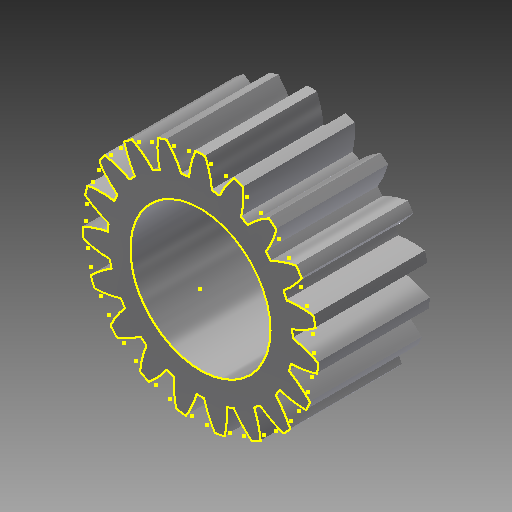
# Autodesk Inventor part: Spur Gear1
Saved by Autodesk Inventor 2017 (Build 210142000, 142)
## iProperties
Created: 2019-09-07
Part Number: Spur Gear1
Material: Steel
Document SubType Name: Modeling
Designer: Dell
Categories: <?xml version="1.0" encoding="UTF-16"?> <MemberInstance><Categories><FamilyTemplate><FamilyTemplateParameter ValueType="xs:double" Id="1" ObjectReferenceKey="da_z" ObjectType="kUserParameterObject"/><FamilyTemplateParameter ValueType="xs:double" Id="2" ObjectReferenceKey="da_b" ObjectType="kUserParameterObject"/><FamilyTemplateParameter ValueType="xs:double" Id="3" ObjectReferenceKey="da_beta" ObjectType="kUserParameterObject"/><FamilyTemplateParameter ValueType="xs:double" Id="4" ObjectReferenceKey="da_da" ObjectType="kUserParameterObject"/><FamilyTemplateParameter ValueType="xs:double" Id="5" ObjectReferenceKey="da_aw" ObjectType="kUserParameterObject"/><FamilyTemplateParameter ValueType="xs:string" Id="6" ObjectReferenceKey="EAIAABAAAACIAQAAAAAAAIAAAAAAAAAA" ObjectType="83910656" SubObjectId="SurfaceGeometry"/></FamilyTemplate><ParamToTemplateMap><ParamToTemplate CategoryParameter="//CategoryParameter[@InternalName='046C89C9-8512-4d59-83FE-43B91F4F132A']" TemplateParameter="1"/><ParamToTemplate CategoryParameter="//CategoryParameter[@InternalName='2552DF32-E462-4b46-AEBF-C6C7768E72AC']" TemplateParameter="2"/><ParamToTemplate CategoryParameter="//CategoryParameter[@InternalName='C9EE641D-15FC-4fae-A226-E94C4372FDD7']" TemplateParameter="3"/><ParamToTemplate><ParamToTemplate CategoryParameter="//CategoryParameter[@InternalName='00B6519A-459B-49c7-AD84-2E56D39A5744']" ConstantValue="0.000000"/></ParamToTemplate><ParamToTemplate><ParamToTemplate CategoryParameter="//CategoryParameter[@InternalName='04B31F0E-C7A6-4894-AA32-9629BEFACF47']" ConstantValue="1.000000"/></ParamToTemplate><ParamToTemplate><ParamToTemplate CategoryParameter="//CategoryParameter[@InternalName='43CBEC2E-7847-49e7-A936-2F7889FCB2D9']" ConstantValue="0.250000"/></ParamToTemplate><ParamToTemplate><ParamToTemplate CategoryParameter="//CategoryParameter[@InternalName='B1EFC894-105D-4ebd-86BF-FA20ED196853']" ConstantValue="0.350000"/></ParamToTemplate><ParamToTemplate><ParamToTemplate CategoryParameter="//CategoryParameter[@InternalName='51175063-3D10-4879-93E8-6246FE8B403D']" ConstantValue="2060000000.000000"/></ParamToTemplate><ParamToTemplate><ParamToTemplate CategoryParameter="//CategoryParameter[@InternalName='A3A52E27-4454-46a9-B0BD-C932399B70AF']" ConstantValue="0.300000"/></ParamToTemplate><ParamToTemplate><ParamToTemplate CategoryParameter="//CategoryParameter[@InternalName='91B76062-C214-41d9-B1B9-14D2AB99603D']" ConstantValue="0.200000"/></ParamToTemplate><ParamToTemplate><ParamToTemplate CategoryParameter="//CategoryParameter[@InternalName='374E806E-8B8A-4dda-A9AA-1039D6500AD2']" ConstantValue="5.000000"/></ParamToTemplate><ParamToTemplate><ParamToTemplate CategoryParameter="//CategoryParameter[@InternalName='2D373A89-B862-43d6-8D0B-0CBF12AB9F6C']" ConstantValue="0.392699"/></ParamToTemplate><ParamToTemplate CategoryParameter="//CategoryParameter[@InternalName='37777632-D6A2-4fac-9D53-DB8ACD95C989']" TemplateParameter="4"/><ParamToTemplate CategoryParameter="//CategoryParameter[@InternalName='FD1017F1-B727-4f7e-9707-0F86F1FF9423']" TemplateParameter="5"/><ParamToTemplate><ParamToTemplate CategoryParameter="//CategoryParameter[@InternalName='9E1B4470-B2D3-4ff1-B813-535BB4CDF51A']" ConstantValue="3520000.000000"/></ParamToTemplate><ParamToTemplate><ParamToTemplate CategoryParameter="//CategoryParameter[@InternalName='F8452263-BFF6-458c-9FB1-07C4B99E95CD']" ConstantValue="11400000.000000"/></ParamToTemplate><ParamToTemplate><ParamToTemplate CategoryParameter="//CategoryParameter[@InternalName='3E3BB259-FD49-497f-8171-6EBC954A3479']" ConstantValue="2.000000"/></ParamToTemplate><ParamToTemplate CategoryParameter="//CategoryParameter[@InternalName='27C3BAF2-7550-4e4b-AE2C-0DB134B7D9B7']" TemplateParameter="6"/></ParamToTemplateMap><Category DisplayName="Gear" InternalName="DC85795E-93AB-48d5-8EEE-5A27447B64BD" Mnemonic="Gear"><CategoryParameter DisplayName="z" InternalName="046C89C9-8512-4d59-83FE-43B91F4F132A" Mnemonic="z"/><CategoryParameter DisplayName="b" InternalName="2552DF32-E462-4b46-AEBF-C6C7768E72AC" Mnemonic="b"/><CategoryParameter DisplayName="||b|" InternalName="C9EE641D-15FC-4fae-A226-E94C4372FDD7" Mnemonic="beta"/><CategoryParameter DisplayName="x" InternalName="00B6519A-459B-49c7-AD84-2E56D39A5744" Mnemonic="x"/><CategoryParameter DisplayName="a*" InternalName="04B31F0E-C7A6-4894-AA32-9629BEFACF47" Mnemonic="a"/><CategoryParameter DisplayName="c*" InternalName="43CBEC2E-7847-49e7-A936-2F7889FCB2D9" Mnemonic="c"/><CategoryParameter DisplayName="r|.f|*" InternalName="B1EFC894-105D-4ebd-86BF-FA20ED196853" Mnemonic="rf"/><CategoryParameter DisplayName="E" InternalName="51175063-3D10-4879-93E8-6246FE8B403D" Mnemonic="E"/><CategoryParameter DisplayName="||m|" InternalName="A3A52E27-4454-46a9-B0BD-C932399B70AF" Mnemonic="mi"/><Category DisplayName="SpurGear" InternalName="26C5A22E-A91E-4dfd-A3B3-23CCAFAE1764" Mnemonic="SpurGear"><CategoryParameter DisplayName="m" InternalName="91B76062-C214-41d9-B1B9-14D2AB99603D" Mnemonic="m"/><CategoryParameter DisplayName="P" InternalName="374E806E-8B8A-4dda-A9AA-1039D6500AD2" Mnemonic="PP"/><CategoryParameter DisplayName="||a|" InternalName="2D373A89-B862-43d6-8D0B-0CBF12AB9F6C" Mnemonic="alpha"/><CategoryParameter DisplayName="d|.a|" InternalName="37777632-D6A2-4fac-9D53-DB8ACD95C989" Mnemonic="da"/><CategoryParameter DisplayName="a|.w|" InternalName="FD1017F1-B727-4f7e-9707-0F86F1FF9423" Mnemonic="aw"/><CategoryParameter DisplayName="||s||.Flim|" InternalName="9E1B4470-B2D3-4ff1-B813-535BB4CDF51A" Mnemonic="sFlim"/><CategoryParameter DisplayName="||s||.Hlim|" InternalName="F8452263-BFF6-458c-9FB1-07C4B99E95CD" Mnemonic="sHlim"/><CategoryParameter DisplayName="type" InternalName="3E3BB259-FD49-497f-8171-6EBC954A3479" Mnemonic="type"/><CategoryParameter DisplayName="PitchDiameter" InternalName="27C3BAF2-7550-4e4b-AE2C-0DB134B7D9B7" Mnemonic="IDS_PITCHDIAM"/></Category></Category></Categories></MemberInstance>
Density: 1 g/cm^3
Appearance: Steel
CustomPartVersion: 1
Author: Dell
Autodesk Inventor part; units mm, degrees
ref_plane "YZ Plane" through (0, 0, 0) normal (1, 0, 0) x (0, 1, 0)
ref_plane "XZ Plane" through (0, 0, 0) normal (0, 1, 0) x (-1, 0, 0)
ref_plane "XY Plane" through (0, 0, 0) normal (0, 0, 1) x (1, 0, 0)
sketch "Sketch1" plane through (0, 0, 0) normal (0, 0, 1) x (1, 0, 0)
  circle A0 centre (0, 0) radius 21
  dimension "d0" = 42
  constraints: 1 centre point
  measures "d0" diameter of A0
extrude "Extrusion1" add sketch "Sketch1" along normal blind 20
ref_plane "Work Plane2" through (0, 0, 10) normal (0, 0, 1) x (1, 0, 0)
sketch "Sketch2" plane through (0, 0, 0) normal (0, 0, -1) x (-1, 0, 0)
  circle A0 centre (0, 0) radius 21 projected
  circle A1 centre (0, 0) radius 19
  dimension "d3" = 38
  constraints: 1 centre point, 1 coincident
  measures "d3" diameter of A1
surface extrude "Pitch Diameter" sketch "Sketch2" against normal through all shown no curves A1
ref_plane "Work Plane8" through (0, 0, 0) normal (0.9863613, 0.1645946, 0) x (0, 0, 1)
ref_plane "Work Plane9" through (0, 0, 0) normal (1, 0, 0) x (0, 1, 0)
spur gear teeth "Spur Gear" teeth 19 pitch diameter 38 tip diameter 42 root diameter 33 face width 20 start plane through (0, 0, 0) normal (0, 0, -1) x (-1, 0, 0)
sketch "Sketch3" plane through (0, 0, 20) normal (0, 0, 1) x (1, 0, 0)
  circle A0 centre (0, 0) radius 12.5
  dimension "d49" = 25
  constraints: 1 centre point, 1 coincident
  measures "d49" diameter of A0
extrude "Extrusion2" cut sketch "Sketch3" against normal through all
sketch "Sketch4" plane through (0, 0, 20) normal (0, 0, 1) x (1, 0, 0)
  circle A0 centre (0, 0) radius 12.5 projected
  arc A1 (-7.6337, 19.5634) -> (-7.2467, 14.8235) centre (8.4724, 18.4924) ccw projected
  arc A2 (-7.2467, 14.8235) -> (-8.4461, 14.1744) centre (0, 0) ccw projected
  arc A3 (-8.4461, 14.1744) -> (-12.2026, 17.0908) centre (-20.1151, 3.0216) ccw projected
  arc A4 (-12.2026, 17.0908) -> (-13.5723, 16.0248) centre (0, 0) ccw projected
  arc A5 (-13.5723, 16.0248) -> (-11.6673, 11.6673) centre (2.0089, 20.2414) ccw projected
  arc A6 (-11.6673, 11.6673) -> (-12.5909, 10.6639) centre (0, 0) ccw projected
  arc A7 (-12.5909, 10.6639) -> (-17.0908, 12.2026) centre (-20.0064, -3.6735) ccw projected
  arc A8 (-17.0908, 12.2026) -> (-18.0401, 10.7496) centre (0, 0) ccw projected
  arc A9 (-18.0401, 10.7496) -> (-14.8235, 7.2467) centre (-4.6724, 19.7969) ccw projected
  arc A10 (-14.8235, 7.2467) -> (-15.3713, 5.9979) centre (0, 0) ccw projected
  arc A11 (-15.3713, 5.9979) -> (-20.127, 5.9921) centre (-17.7296, -9.9705) ccw projected
  arc A12 (-20.127, 5.9921) -> (-20.5531, 4.3095) centre (0, 0) ccw projected
  arc A13 (-20.5531, 4.3095) -> (-16.3733, 2.0409) centre (-10.8472, 17.2072) ccw projected
  arc A14 (-16.3733, 2.0409) -> (-16.4859, 0.6819) centre (0, 0) ccw projected
  arc A15 (-16.4859, 0.6819) -> (-20.9821, -0.8678) centre (-13.5315, -15.1871) ccw projected
  arc A16 (-20.9821, -0.8678) -> (-20.8387, -2.5975) centre (0, 0) ccw projected
  arc A17 (-20.8387, -2.5975) -> (-16.1488, -3.3861) centre (-15.8467, 12.7527) ccw projected
  arc A18 (-16.1488, -3.3861) -> (-15.8141, -4.708) centre (0, 0) ccw projected
  arc A19 (-15.8141, -4.708) -> (-19.5634, -7.6337) centre (-7.8671, -18.7579) ccw projected
  arc A20 (-19.5634, -7.6337) -> (-18.8662, -9.2231) centre (0, 0) ccw projected
  arc A21 (-18.8662, -9.2231) -> (-14.1744, -8.4461) centre (-19.1289, 6.9163) ccw projected
  arc A22 (-14.1744, -8.4461) -> (-13.4285, -9.5878) centre (0, 0) ccw projected
  arc A23 (-13.4285, -9.5878) -> (-16.0248, -13.5723) centre (-1.3502, -20.296) ccw projected
  arc A24 (-16.0248, -13.5723) -> (-14.8492, -14.8492) centre (0, 0) ccw projected
  arc A25 (-14.8492, -14.8492) -> (-10.6639, -12.5909) centre (-20.3381, 0.3305) ccw projected
  arc A26 (-10.6639, -12.5909) -> (-9.5878, -13.4285) centre (0, 0) ccw projected
  arc A27 (-9.5878, -13.4285) -> (-10.7496, -18.0401) centre (5.3131, -19.6347) ccw projected
  arc A28 (-10.7496, -18.0401) -> (-9.2231, -18.8662) centre (0, 0) ccw projected
  arc A29 (-9.2231, -18.8662) -> (-5.9979, -15.3713) centre (-19.3435, -6.2912) ccw projected
  arc A30 (-5.9979, -15.3713) -> (-4.708, -15.8141) centre (0, 0) ccw projected
  arc A31 (-4.708, -15.8141) -> (-4.3095, -20.5531) centre (11.4006, -16.8457) ccw projected
  arc A32 (-4.3095, -20.5531) -> (-2.5975, -20.8387) centre (0, 0) ccw projected
  arc A33 (-2.5975, -20.8387) -> (-0.6819, -16.4859) centre (-16.2526, -12.2312) ccw projected
  arc A34 (-0.6819, -16.4859) -> (0.6819, -16.4859) centre (0, 0) ccw projected
  arc A35 (0.6819, -16.4859) -> (2.5975, -20.8387) centre (16.2526, -12.2312) ccw projected
  arc A36 (2.5975, -20.8387) -> (4.3095, -20.5531) centre (0, 0) ccw projected
  arc A37 (4.3095, -20.5531) -> (4.708, -15.8141) centre (-11.4006, -16.8457) ccw projected
  arc A38 (4.708, -15.8141) -> (5.9979, -15.3713) centre (0, 0) ccw projected
  arc A39 (5.9979, -15.3713) -> (9.2231, -18.8662) centre (19.3435, -6.2912) ccw projected
  arc A40 (9.2231, -18.8662) -> (10.7496, -18.0401) centre (0, 0) ccw projected
  arc A41 (10.7496, -18.0401) -> (9.5878, -13.4285) centre (-5.3131, -19.6347) ccw projected
  arc A42 (9.5878, -13.4285) -> (10.6639, -12.5909) centre (0, 0) ccw projected
  arc A43 (10.6639, -12.5909) -> (14.8492, -14.8492) centre (20.3381, 0.3305) ccw projected
  arc A44 (14.8492, -14.8492) -> (16.0248, -13.5723) centre (0, 0) ccw projected
  arc A45 (16.0248, -13.5723) -> (13.4285, -9.5878) centre (1.3502, -20.296) ccw projected
  arc A46 (13.4285, -9.5878) -> (14.1744, -8.4461) centre (0, 0) ccw projected
  arc A47 (14.1744, -8.4461) -> (18.8662, -9.2231) centre (19.1289, 6.9163) ccw projected
  arc A48 (18.8662, -9.2231) -> (19.5634, -7.6337) centre (0, 0) ccw projected
  arc A49 (19.5634, -7.6337) -> (15.8141, -4.708) centre (7.8671, -18.7579) ccw projected
  arc A50 (15.8141, -4.708) -> (16.1488, -3.3861) centre (0, 0) ccw projected
  arc A51 (16.1488, -3.3861) -> (20.8387, -2.5975) centre (15.8467, 12.7527) ccw projected
  arc A52 (20.8387, -2.5975) -> (20.9821, -0.8678) centre (0, 0) ccw projected
  arc A53 (20.9821, -0.8678) -> (16.4859, 0.6819) centre (13.5315, -15.1871) ccw projected
  arc A54 (16.4859, 0.6819) -> (16.3733, 2.0409) centre (0, 0) ccw projected
  arc A55 (16.3733, 2.0409) -> (20.5531, 4.3095) centre (10.8472, 17.2072) ccw projected
  arc A56 (20.5531, 4.3095) -> (20.127, 5.9921) centre (0, 0) ccw projected
  arc A57 (20.127, 5.9921) -> (15.3713, 5.9979) centre (17.7296, -9.9705) ccw projected
  arc A58 (15.3713, 5.9979) -> (14.8235, 7.2467) centre (0, 0) ccw projected
  arc A59 (14.8235, 7.2467) -> (18.0401, 10.7496) centre (4.6724, 19.7969) ccw projected
  arc A60 (18.0401, 10.7496) -> (17.0908, 12.2026) centre (0, 0) ccw projected
  arc A61 (17.0908, 12.2026) -> (12.5909, 10.6639) centre (20.0064, -3.6735) ccw projected
  arc A62 (12.5909, 10.6639) -> (11.6673, 11.6673) centre (0, 0) ccw projected
  arc A63 (11.6673, 11.6673) -> (13.5723, 16.0248) centre (-2.0089, 20.2414) ccw projected
  arc A64 (13.5723, 16.0248) -> (12.2026, 17.0908) centre (0, 0) ccw projected
  arc A65 (12.2026, 17.0908) -> (8.4461, 14.1744) centre (20.1151, 3.0216) ccw projected
  arc A66 (8.4461, 14.1744) -> (7.2467, 14.8235) centre (0, 0) ccw projected
  arc A67 (7.2467, 14.8235) -> (7.6337, 19.5634) centre (-8.4724, 18.4924) ccw projected
  arc A68 (7.6337, 19.5634) -> (5.9921, 20.127) centre (0, 0) ccw projected
  arc A69 (5.9921, 20.127) -> (3.3861, 16.1488) centre (18.0441, 9.3892) ccw projected
  arc A70 (3.3861, 16.1488) -> (2.0409, 16.3733) centre (0, 0) ccw projected
  arc A71 (2.0409, 16.3733) -> (0.8678, 20.9821) centre (-14.0178, 14.7394) ccw projected
  arc A72 (0.8678, 20.9821) -> (-0.8678, 20.9821) centre (0, 0) ccw projected
  arc A73 (-0.8678, 20.9821) -> (-2.0409, 16.3733) centre (14.0178, 14.7394) ccw projected
  arc A74 (-2.0409, 16.3733) -> (-3.3861, 16.1488) centre (0, 0) ccw projected
  arc A75 (-3.3861, 16.1488) -> (-5.9921, 20.127) centre (-18.0441, 9.3892) ccw projected
  arc A76 (-5.9921, 20.127) -> (-7.6337, 19.5634) centre (0, 0) ccw projected
equation "\"d0\" = da_da"
equation "\"d1\" = da_b"
equation "\"d3\" = da_dw"
equation "\"d16\" = da_aw"
equation "\"d43\" = da_aw"
equation "\"d46\" = da_aw"
equation "\"da_da\" = 42"
equation "\"da_b\" = 20"
equation "\"da_dw\" = 38"
equation "\"da_aw\" = 28"
body "Solid1"
body "Srf1"
